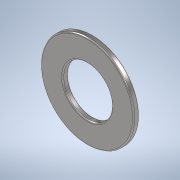
# Autodesk Inventor part: M4 SHim
Saved by Autodesk Inventor 2020 (Build 240168000, 168)
## iProperties
Created: 2023-06-16
Part Number: M4 SHim
Material: Stainless Steel
Document SubType Name: Modeling
Designer: Ishaan
Density: 8 g/cm^3
Appearance: Semi-Polished
Author: Ishaan
Autodesk Inventor part; units mm, degrees
ref_plane "YZ Plane" through (0, 0, 0) normal (1, 0, 0) x (0, 1, 0)
ref_plane "XZ Plane" through (0, 0, 0) normal (0, 1, 0) x (-1, 0, 0)
ref_plane "XY Plane" through (0, 0, 0) normal (0, 0, 1) x (1, 0, 0)
sketch "Sketch1" plane through (0, 0, 0) normal (0, 0, 1) x (1, 0, 0)
  circle A0 centre (0, 0) radius 2.1
  circle A1 centre (0, 0) radius 4
  dimension "d0" = 4.2
  dimension "d1" = 8
  constraints: 2 centre point, 2 coincident
  measures "d0" diameter of A0
  measures "d1" diameter of A1
extrude "Extrusion1" add sketch "Sketch1" along normal mid plane 0.5
fillet "Fillet1" radius 0.1 4 edges at (-2.1, 0, -0.25) (-2.1, 0, 0.25) (-4, 0, 0.25) (-4, 0, -0.25)
body "Solid1"
